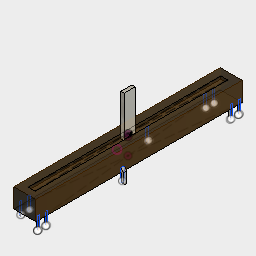
slidepot v1 (Autodesk Fusion 360 design; units mm, degrees)
Autodesk Fusion 360 part; units mm, degrees
sketch "Sketch1" plane through (0, 0, 0) normal (0, 1, 0) x (1, 0, 0)
  line L0 (4, 37.5) -> (-4, 37.5)
  line L1 (-4, 37.5) -> (-4, -37.5)
  line L2 (-4, -37.5) -> (4, -37.5)
  line L3 (4, -37.5) -> (4, 37.5)
  line L4 (4, 37.5) -> (-4, -37.5) construction
  line L5 (-4, 37.5) -> (4, -37.5) construction
  dimension "d1" = 75
  dimension "d2" = 8
  measures "d1" distance of L0.end L1.end
  measures "d2" distance of L1.end L2.end
extrude "Extrude1" add sketch "Sketch1" along normal blind 7
sketch "Sketch2" plane through (0, 7, 0) normal (0, 1, 0) x (-1, 0, 0)
  line L0 (-4, 37.5) -> (-4, -37.5)
  line L1 (-4, -37.5) -> (4, -37.5)
  line L2 (4, -37.5) -> (4, 37.5)
  line L3 (4, 37.5) -> (-4, 37.5)
  line L4 (-1.25, -35) -> (1.25, -35)
  line L5 (1.25, -35) -> (1.25, 35)
  line L6 (1.25, 35) -> (-1.25, 35)
  line L7 (-1.25, 35) -> (-1.25, -35)
  line L8 (-1.25, -35) -> (1.25, 35) construction
  line L9 (1.25, -35) -> (-1.25, 35) construction
  dimension "d5" = 70
  dimension "d6" = 2.5
  measures "d5" distance of L4.end L5.end
  measures "d6" distance of L5.end L6.end
extrude "Extrude2" cut sketch "Sketch2" against normal blind 1 contours L4 L5 L6 L7
sketch "Sketch3" plane through (4, 0, 0) normal (1, 0, 0) x (0, 0, -1)
  line L0 (-37.5, 0) -> (37.5, 0)
  line L1 (37.5, 0) -> (37.5, 7)
  line L2 (37.5, 7) -> (-37.5, 7)
  line L3 (-37.5, 7) -> (-37.5, 0)
  line L4 (36.9, 1.5) -> (36.1, 1.5)
  line L5 (36.9, 1.5) -> (36.9, -3.1)
  line L6 (36.1, -3.1) -> (36.1, 1.5)
  line L7 (33.9, 1.5) -> (33.1, 1.5)
  line L8 (33.9, 1.5) -> (33.9, -3.1)
  line L9 (33.1, -3.1) -> (33.1, 1.5)
  line L10 (-36.9, -3.1) -> (-36.9, 1.5)
  line L11 (-36.1, 1.5) -> (-36.9, 1.5)
  line L12 (-36.1, 1.5) -> (-36.1, -3.1)
  line L13 (-33.1, 1.5) -> (-33.9, 1.5)
  line L14 (-33.1, 1.5) -> (-33.1, -3.1)
  line L15 (-33.9, -3.1) -> (-33.9, 1.5)
  arc A0 (-36.9, -3.1) -> (-36.1, -3.1) centre (-36.5, -3.1) ccw
  arc A1 (-33.9, -3.1) -> (-33.1, -3.1) centre (-33.5, -3.1) ccw
  arc A2 (33.1, -3.0992) -> (33.9, -3.1) centre (33.5, -3.1) ccw
  arc A3 (36.1, -3.1) -> (36.9, -3.1) centre (36.5, -3.1) ccw
  dimension "d18" = 1.5
  dimension "d19" = 0.5
  dimension "d20" = 0.8
  dimension "d21" = 0.8
  dimension "d22" = 0.8
  dimension "d23" = 0.8
  dimension "d24" = 73.2
  dimension "d25" = 67
  dimension "d26" = 3
  dimension "d27" = 3
  measures "d20" distance of L10 L12
  measures "d21" distance of L14 L15
  measures "d22" distance of L8 L9
  measures "d23" distance of L5 L6
  measures "d25" distance of A1.centre A2.centre
  measures "d26" distance of A0.centre A1.centre
  measures "d27" distance of A2.centre A3.centre
sketch "Sketch4" plane through (-4, 0, 0) normal (-1, 0, 0) x (0, 0, 1)
  line L0 (-37.5, 0) -> (37.5, 0)
  line L1 (37.5, 0) -> (37.5, 7)
  line L2 (37.5, 7) -> (-37.5, 7)
  line L3 (-37.5, 7) -> (-37.5, 0)
  line L4 (-32.4, -3.1) -> (-32.4, 1.5)
  line L5 (-31.6, 1.5) -> (-32.4, 1.5)
  line L6 (-31.6, 1.5) -> (-31.6, -3.1)
  line L7 (-35.4, -3.1) -> (-35.4, 1.5)
  line L8 (-34.6, 1.5) -> (-35.4, 1.5)
  line L9 (-34.6, 1.5) -> (-34.6, -3.1)
  line L10 (31.6, -3.1) -> (31.6, 1.5)
  line L11 (32.4, 1.5) -> (31.6, 1.5)
  line L12 (32.4, 1.5) -> (32.4, -3.1)
  line L13 (35.4, 1.5) -> (34.6, 1.5)
  line L14 (35.4, 1.5) -> (35.4, -3.1)
  line L15 (34.6, -3.1) -> (34.6, 1.5)
  arc A0 (31.6, -3.1) -> (32.4, -3.1) centre (32, -3.1) ccw
  arc A1 (34.6, -3.1) -> (35.4, -3.1) centre (35, -3.1) ccw
  arc A2 (-32.4, -3.1) -> (-31.6, -3.1) centre (-32, -3.1) ccw
  arc A3 (-35.4, -3.1) -> (-34.6, -3.1) centre (-35, -3.1) ccw
  dimension "d12" = 3
  dimension "d13" = 1
  dimension "d28" = 0.8
  dimension "d29" = 0.8
  dimension "d30" = 0.8
  dimension "d31" = 0.8
  dimension "d32" = 3
  dimension "d33" = 3.2
  dimension "d34" = 70.2
  dimension "d35" = 64
  measures "d28" distance of L7 L9
  measures "d29" distance of L4 L6
  measures "d30" distance of L10 L12
  measures "d31" distance of L14 L15
  measures "d32" distance of A2.centre A3.centre
  measures "d35" distance of A0.centre A2.centre
extrude "Extrude3" add sketch "Sketch4" against normal blind 0.4 contours L0 L7 L9 A3 | L0 L4 L6 A2 | L0 L14 L15 A1 | L0 L10 L12 A0
extrude "Extrude4" add sketch "Sketch3" against normal blind 0.4 contours L0 L10 L12 A0 | L0 L14 L15 A1 | L0 L5 L6 A3 | L0 L8 L9 A2
sketch "Sketch5" plane through (4, 0, 0) normal (1, 0, 0) x (0, 0, -1)
  line L0 (-37.5, 0) -> (-36.9, 0)
  line L1 (-36.9, 0) -> (-36.9, -3.1)
  arc A0 (-36.9, -3.1) -> (-36.1, -3.1) centre (-36.5, -3.1) ccw
  line L2 (-36.1, -3.1) -> (-36.1, 0)
  line L3 (-36.1, 0) -> (-33.9, 0)
  line L4 (-33.9, 0) -> (-33.9, -3.1)
  arc A1 (-33.9, -3.1) -> (-33.1, -3.1) centre (-33.5, -3.1) ccw
  line L5 (-33.1, -3.1) -> (-33.1, 0)
  line L6 (-33.1, 0) -> (33.1, 0)
  line L7 (33.1, 0) -> (33.1, -3.0992)
  arc A2 (33.1, -3.0992) -> (33.9, -3.1) centre (33.5, -3.1) ccw
  line L8 (33.9, -3.1) -> (33.9, 0)
  line L9 (33.9, 0) -> (36.1, 0)
  line L10 (36.1, 0) -> (36.1, -3.1)
  arc A3 (36.1, -3.1) -> (36.9, -3.1) centre (36.5, -3.1) ccw
  line L11 (36.9, -3.1) -> (36.9, 0)
  line L12 (36.9, 0) -> (37.5, 0)
  line L13 (37.5, 0) -> (37.5, 7)
  line L14 (37.5, 7) -> (-37.5, 7)
  line L15 (-37.5, 7) -> (-37.5, 0)
  line L16 (-6.6, 1.5) -> (-5.4, 1.5)
  line L17 (-5.4, 1.5) -> (-5.4, -2.9)
  line L18 (-6.6, -2.9) -> (-6.6, 1.5)
  arc A4 (-6.6, -2.9) -> (-5.4, -2.9) centre (-6, -2.9) ccw
  dimension "d40" = 1.2
  dimension "d42" = 6
  measures "d40" distance of L16.start L16.end
  measures "d42" distance of origin A4.centre
extrude "Extrude5" add sketch "Sketch5" along normal blind 1 contours L6 L16 L17 L18 | L6 L17 L18 A4
sketch "Sketch6" plane through (-4, 0, 0) normal (-1, 0, 0) x (0, 0, 1)
  line L0 (-37.5, 0) -> (-35.4, 0)
  line L1 (-35.4, 0) -> (-35.4, -3.1)
  arc A0 (-35.4, -3.1) -> (-34.6, -3.1) centre (-35, -3.1) ccw
  line L2 (-34.6, -3.1) -> (-34.6, 0)
  line L3 (-34.6, 0) -> (-32.4, 0)
  line L4 (-32.4, 0) -> (-32.4, -3.1)
  arc A1 (-32.4, -3.1) -> (-31.6, -3.1) centre (-32, -3.1) ccw
  line L5 (-31.6, -3.1) -> (-31.6, 0)
  line L6 (-31.6, 0) -> (31.6, 0)
  line L7 (31.6, 0) -> (31.6, -3.1)
  arc A2 (31.6, -3.1) -> (32.4, -3.1) centre (32, -3.1) ccw
  line L8 (32.4, -3.1) -> (32.4, 0)
  line L9 (32.4, 0) -> (34.6, 0)
  line L10 (34.6, 0) -> (34.6, -3.1)
  arc A3 (34.6, -3.1) -> (35.4, -3.1) centre (35, -3.1) ccw
  line L11 (35.4, -3.1) -> (35.4, 0)
  line L12 (35.4, 0) -> (37.5, 0)
  line L13 (37.5, 0) -> (37.5, 7)
  line L14 (37.5, 7) -> (-37.5, 7)
  line L15 (-37.5, 7) -> (-37.5, 0)
  line L16 (-11.6, 1.5) -> (-10.4, 1.5)
  line L17 (-10.4, 1.5) -> (-10.4, -2.9)
  line L18 (-11.6, -2.9) -> (-11.6, 1.5)
  arc A4 (-11.6, -2.9) -> (-10.4, -2.9) centre (-11, -2.9) ccw
  dimension "d55" = 11
  measures "d55" distance of A4.centre origin
extrude "Extrude6" add sketch "Sketch6" along normal blind 1 contours L6 L16 L17 L18 | L6 L17 L18 A4
chamfer "Chamfer1" distance 1 angle 45 1 edges at (-5, 1.5, -11)
chamfer "Chamfer2" distance 1 angle 45 1 edges at (5, 1.5, 6)
move_face "OffsetFaces1" offset -0.4 1 faces at (4, -1.9333, 6.2)
move_face "OffsetFaces2" offset -0.4 1 faces at (-4, -0.9667, -11.2)
sketch "Sketch7" plane through (0, 6, 0) normal (0, 1, 0) x (-1, 0, 0)
  line L0 (-1.25, 35) -> (-1.25, -35)
  line L1 (-1.25, -35) -> (1.25, -35)
  line L2 (1.25, -35) -> (1.25, 35)
  line L3 (1.25, 35) -> (-1.25, 35)
  line L4 (-0.6, -2) -> (0.6, -2)
  line L5 (0.6, -2) -> (0.6, 2)
  line L6 (0.6, 2) -> (-0.6, 2)
  line L7 (-0.6, 2) -> (-0.6, -2)
  line L8 (-0.6, -2) -> (0.6, 2) construction
  line L9 (0.6, -2) -> (-0.6, 2) construction
  dimension "d51" = 1.2
  dimension "d52" = 4
  measures "d51" distance of L5.end L6.end
  measures "d52" distance of L4.end L5.end
extrude "Extrude7" add sketch "Sketch7" along normal blind 15 contours L4 L5 L6 L7
